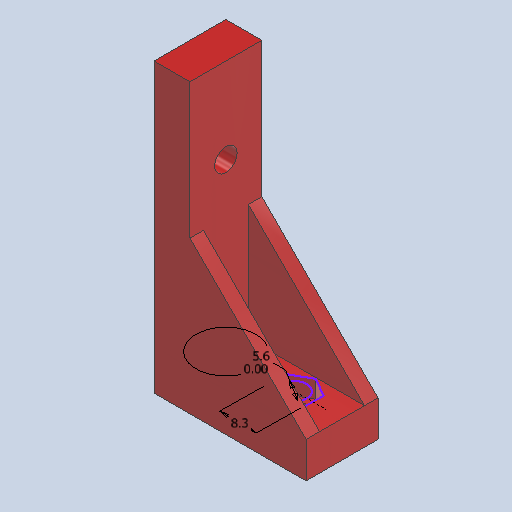
# Autodesk Inventor part: Lower Limit Switch
Saved by Autodesk Inventor 2022 (Build 260153000, 153)
## iProperties
Created: 2022-10-20
Part Number: Lower Limit Switch
Material: Generic
Document SubType Name: Modeling
Designer: matt
Density: 1 g/cm^3
Appearance: Default
Author: matt
Autodesk Inventor part; units mm, degrees
ref_plane "YZ Plane" through (0, 0, 0) normal (1, 0, 0) x (0, 1, 0)
ref_plane "XZ Plane" through (0, 0, 0) normal (0, 1, 0) x (-1, 0, 0)
ref_plane "XY Plane" through (0, 0, 0) normal (0, 0, 1) x (1, 0, 0)
sketch "Sketch1" plane through (0, 0, 0) normal (0, 0, 1) x (1, 0, 0)
  line L0 (0, 64) -> (0, 0)
  line L1 (24.8907, 0) -> (21.3073, 0)
  line L2 (0, 64) -> (8, 64)
  line L3 (33.8546, 8) -> (33.8546, 0)
  line L4 (33.8546, 0) -> (0, 0)
  line L5 (0, 0) -> (0, 64)
  line L6 (8, 64) -> (8, 8)
  line L7 (8, 8) -> (33.8546, 8)
  line L8 (33.8546, 8) -> (8, 33.8546)
  line L9 (33.8546, 8) -> (70.4186, 8) construction
  point P0 (0, 0)
  dimension "d0" = 8
  dimension "d1" = 8
  dimension "d2" = 135
  dimension "d9" = 64
  constraints: 20 end point, 2 horizontal, 2 parallel, 2 perpendicular, 1 equal length, 1 point on line, 1 vertical
  measures "d0" distance between parallel lines of L4 L7
  measures "d1" distance between parallel lines of L6 L0
  measures "d2" angle of L9 L8
  measures "d9" distance between parallel lines of L4 L2
extrude "Extrusion1" add sketch "Sketch1" along normal blind 3
extrude "Extrusion2" add sketch "Sketch1" against normal blind 10 contours L2 L6 L7 L3 L4 L1 L0
extrude "Extrusion3" add sketch "Sketch1" against normal blind 3 from surface at -10
sketch "Sketch2" plane through (8, 33.8546, 3) normal (1, 0, 0) x (0, 0, -1)
  circle A0 centre (8, 11.1454) radius 2.5
  circle A1 centre (8, -20.8546) radius 2.5
  line L0 (16, 30.1454) -> (0, 30.1454) projected
  line L1 (8, 30.1454) -> (8, -25.8546) construction
  line L2 (3, -25.8546) -> (13, -25.8546) construction
  point P0 (3, -33.8546)
  dimension "d20" = 32
  dimension "d21" = 19
  constraints: 2 centre point, 2 end point, 2 midpoint, 2 point on line
  measures "d20" distance of A1.centre A0.centre
  measures "d21" distance from line of L0 A0.centre
extrude "Extrusion4" cut sketch "Sketch2" against normal through all
sketch "Sketch3" plane through (8, 8, 0) normal (0, 1, 0) x (1, 0, 0)
  circle A0 centre (15.0917, 5) radius 2.8
  line L0 (0, 0) -> (0, 10) projected
  line L1 (0, 7.5) -> (0, 2.5) construction
  line L2 (0, 5) -> (22.225, 5) construction
  line L3 (0, 5) -> (22.225, 5) construction
  line L4 (10.9735, 7.4504) -> (15.1547, 9.7916)
  line L5 (15.1547, 9.7916) -> (19.2728, 7.3412)
  line L6 (19.2728, 7.3412) -> (19.2098, 2.5496)
  line L7 (19.2098, 2.5496) -> (15.0287, 0.2084)
  line L8 (15.0287, 0.2084) -> (10.9105, 2.6588)
  line L9 (10.9105, 2.6588) -> (10.9735, 7.4504)
  point P0 (-8, 0)
  dimension "d13" = 5.6
  dimension "d14" = 0
  dimension "d22" = 8.3
  constraints: 16 end point, 1 centre point, 1 coincident, 1 collinear, 1 horizontal, 1 midpoint, 1 point on line, 13 other
  measures "d13" diameter of A0
  measures "d14" distance between parallel lines of L2 L3
  measures "d22" distance between parallel lines of L6 L9
extrude "Extrusion5" cut sketch "Sketch3" against normal through all contours A0
extrude "Extrusion7" cut sketch "Sketch3" against normal blind 4 contours A0 | L4 L5 L6 L7 L8 L9
equation "\"d1\" = d0"
body "Solid1"
